Autodesk Fusion 360 part; units mm, degrees
(part 2 of 8)
  spline S328 degree 3 poles (150.3469, -208.3577) (147.0321, -208.3577) (145.9386, -207.6875) (144.7041, -207.6875) knots 0 0 0 0 1 1 1 1
  spline S329 degree 3 poles (144.7041, -207.6875) (143.8199, -207.6875) (143.538, -208.0049) (142.9741, -208.0049) knots 0 0 0 0 1 1 1 1
  spline S330 degree 3 poles (142.9741, -208.0049) (142.517, -208.0049) (142.2351, -207.5816) (142.0557, -206.9114) knots 0 0 0 0 1 1 1 1
  spline S331 degree 3 poles (142.0557, -206.9114) (141.9147, -206.3821) (140.787, -201.1963) (140.787, -200.9144) knots 0 0 0 0 1 1 1 1
  spline S332 degree 3 poles (140.787, -200.9144) (140.787, -200.632) (141.5644, -199.8913) (141.9873, -199.8913) knots 0 0 0 0 1 1 1 1
  spline S333 degree 3 poles (141.9873, -199.8913) (142.658, -199.8913) (145.6225, -205.8178) (150.7356, -205.8178) knots 0 0 0 0 1 1 1 1
  spline S334 degree 3 poles (150.7356, -205.8178) (152.7818, -205.8178) (154.0889, -204.9007) (154.0889, -203.4189) knots 0 0 0 0 1 1 1 1
  spline S335 degree 3 poles (154.0889, -203.4189) (154.0504, -199.3621) (141.4918, -199.9618) (141.4918, -191.1422) knots 0 0 0 0 1 1 1 1
  spline S336 degree 3 poles (177.5118, -204.8653) (177.5118, -206.3823) (179.4524, -206.2764) (179.4524, -206.8059) knots 0 0 0 0 1 1 1 1
  spline S337 degree 3 poles (179.4524, -206.8059) (179.4524, -207.2291) (179.0625, -208.0053) (178.7789, -208.0053) knots 0 0 0 0 1 1 1 1
  spline S338 degree 3 poles (178.7789, -208.0053) (177.4054, -207.9344) (175.6774, -207.8994) (173.9495, -207.8994) knots 0 0 0 0 1 1 1 1
  spline S339 degree 3 poles (173.9495, -207.8994) (172.2171, -207.8994) (170.5245, -207.9344) (169.1156, -208.0053) knots 0 0 0 0 1 1 1 1
  spline S340 degree 3 poles (169.1156, -208.0053) (168.832, -208.0053) (168.4775, -207.2291) (168.4775, -206.8059) knots 0 0 0 0 1 1 1 1
  spline S341 degree 3 poles (168.4775, -206.8059) (168.4775, -206.2765) (170.3827, -206.3823) (170.3827, -204.8653) knots 0 0 0 0 1 1 1 1
  line L72 (170.3827, -204.8653) -> (170.3827, -187.6147)
  spline S342 degree 3 poles (170.3827, -187.6147) (170.3827, -187.0853) (169.9618, -186.8385) (169.0092, -186.8385) knots 0 0 0 0 1 1 1 1
  spline S343 degree 3 poles (169.0092, -186.8385) (164.9507, -186.8385) (163.2582, -191.6715) (162.5891, -191.6715) knots 0 0 0 0 1 1 1 1
  spline S344 degree 3 poles (162.5891, -191.6715) (162.1638, -191.6715) (161.3884, -191.3188) (161.3884, -191.0011) knots 0 0 0 0 1 1 1 1
  spline S345 degree 3 poles (161.3884, -191.0011) (161.3884, -190.7189) (162.0574, -185.8154) (162.1283, -185.3568) knots 0 0 0 0 1 1 1 1
  spline S346 degree 3 poles (162.1283, -185.3568) (162.2701, -184.4397) (162.6246, -184.2243) (163.3645, -184.2633) knots 0 0 0 0 1 1 1 1
  spline S347 degree 3 poles (163.3645, -184.2633) (167.0331, -184.3338) (170.6663, -184.3692) (174.2995, -184.3692) knots 0 0 0 0 1 1 1 1
  spline S348 degree 3 poles (174.2995, -184.3692) (177.9327, -184.3692) (181.6058, -184.3338) (185.2389, -184.2633) knots 0 0 0 0 1 1 1 1
  spline S349 degree 3 poles (185.2389, -184.2633) (185.9434, -184.2244) (186.3688, -184.4397) (186.3688, -185.0746) knots 0 0 0 0 1 1 1 1
  spline S350 degree 3 poles (186.3688, -185.0746) (186.3688, -185.8154) (185.8415, -190.7189) (185.8415, -191.0011) knots 0 0 0 0 1 1 1 1
  spline S351 degree 3 poles (185.8415, -191.0011) (185.8415, -191.2834) (185.0617, -191.6715) (184.6408, -191.6715) knots 0 0 0 0 1 1 1 1
  spline S352 degree 3 poles (184.6408, -191.6715) (183.9718, -191.6715) (183.6882, -186.8385) (178.6416, -186.8385) knots 0 0 0 0 1 1 1 1
  spline S353 degree 3 poles (178.6416, -186.8385) (177.9327, -186.8385) (177.5118, -186.7326) (177.5118, -187.6147) knots 0 0 0 0 1 1 1 1
  line L73 (177.5118, -187.6147) -> (177.5118, -204.8653)
  spline S354 degree 3 poles (199.0684, -208.3577) (192.9284, -208.3577) (189.4714, -204.8651) (189.4714, -198.48) knots 0 0 0 0 1 1 1 1
  line L74 (189.4714, -198.48) -> (189.4714, -187.3674)
  spline S355 degree 3 poles (189.4714, -187.3674) (189.4714, -185.8857) (187.5667, -185.9915) (187.5667, -185.4274) knots 0 0 0 0 1 1 1 1
  spline S356 degree 3 poles (187.5667, -185.4274) (187.5667, -185.0039) (187.9192, -184.263) (188.2352, -184.263) knots 0 0 0 0 1 1 1 1
  spline S357 degree 3 poles (188.2352, -184.263) (189.65, -184.3336) (191.3395, -184.3688) (193.0703, -184.3688) knots 0 0 0 0 1 1 1 1
  spline S358 degree 3 poles (193.0703, -184.3688) (194.7644, -184.3688) (196.4906, -184.3336) (197.8688, -184.263) knots 0 0 0 0 1 1 1 1
  spline S359 degree 3 poles (197.8688, -184.263) (198.1481, -184.263) (198.5373, -185.0039) (198.5373, -185.4274) knots 0 0 0 0 1 1 1 1
  spline S360 degree 3 poles (198.5373, -185.4274) (198.5373, -185.9915) (196.5959, -185.8857) (196.5959, -187.3674) knots 0 0 0 0 1 1 1 1
  line L75 (196.5959, -187.3674) -> (196.5959, -198.9031)
  spline S361 degree 3 poles (196.5959, -198.9031) (196.5959, -202.9956) (198.3632, -205.1123) (201.3578, -205.1123) knots 0 0 0 0 1 1 1 1
  spline S362 degree 3 poles (201.3578, -205.1123) (204.3568, -205.1123) (206.1242, -202.9956) (206.1242, -198.9031) knots 0 0 0 0 1 1 1 1
  line L76 (206.1242, -198.9031) -> (206.1242, -187.3674)
  spline S363 degree 3 poles (206.1242, -187.3674) (206.1242, -185.8857) (204.1828, -185.9915) (204.1828, -185.4274) knots 0 0 0 0 1 1 1 1
  spline S364 degree 3 poles (204.1828, -185.4274) (204.1828, -185.0039) (204.572, -184.2241) (204.8513, -184.263) knots 0 0 0 0 1 1 1 1
  spline S365 degree 3 poles (204.8513, -184.263) (205.5564, -184.3336) (206.4767, -184.3688) (207.3925, -184.3688) knots 0 0 0 0 1 1 1 1
  spline S366 degree 3 poles (207.3925, -184.3688) (208.3082, -184.3688) (209.2285, -184.3336) (209.9337, -184.263) knots 0 0 0 0 1 1 1 1
  spline S367 degree 3 poles (209.9337, -184.263) (210.213, -184.2241) (210.4969, -185.0039) (210.4969, -185.4274) knots 0 0 0 0 1 1 1 1
  spline S368 degree 3 poles (210.4969, -185.4274) (210.4969, -185.9915) (208.6608, -185.8857) (208.6608, -187.3674) knots 0 0 0 0 1 1 1 1
  line L77 (208.6608, -187.3674) -> (208.6608, -198.48)
  spline S369 degree 3 poles (208.6608, -198.48) (208.6608, -204.8651) (205.2039, -208.3577) (199.0683, -208.3577) knots 0 0 0 0 1 1 1 1
  spline S370 degree 3 poles (213.773, -187.4032) (213.28, -185.9921) (211.6589, -186.0272) (211.6589, -185.4631) knots 0 0 0 0 1 1 1 1
  spline S371 degree 3 poles (211.6589, -185.4631) (211.6589, -185.0398) (212.0476, -184.2989) (212.3272, -184.2989) knots 0 0 0 0 1 1 1 1
  spline S372 degree 3 poles (212.3272, -184.2989) (213.7398, -184.3695) (215.5743, -184.4008) (217.4087, -184.4008) knots 0 0 0 0 1 1 1 1
  spline S373 degree 3 poles (217.4087, -184.4008) (219.2432, -184.4008) (221.0776, -184.3695) (222.4854, -184.2989) knots 0 0 0 0 1 1 1 1
  spline S374 degree 3 poles (222.4854, -184.2989) (222.7698, -184.2989) (223.1206, -185.0398) (223.1206, -185.4631) knots 0 0 0 0 1 1 1 1
  spline S375 degree 3 poles (223.1206, -185.4631) (223.1206, -186.0272) (220.9022, -185.9921) (221.3952, -187.4032) knots 0 0 0 0 1 1 1 1
  line L78 (226.652, -202.5727) -> (231.9089, -187.4032)
  spline S376 degree 3 poles (231.9089, -187.4032) (232.4019, -185.9921) (230.1787, -186.0272) (230.1787, -185.4631) knots 0 0 0 0 1 1 1 1
  spline S377 degree 3 poles (230.1787, -185.4631) (230.1787, -185.0398) (230.5295, -184.2633) (230.8139, -184.2989) knots 0 0 0 0 1 1 1 1
  spline S378 degree 3 poles (230.8139, -184.2989) (231.378, -184.3695) (232.4351, -184.4008) (233.4921, -184.4008) knots 0 0 0 0 1 1 1 1
  spline S379 degree 3 poles (233.4921, -184.4008) (234.554, -184.4008) (235.611, -184.3695) (236.1419, -184.2989) knots 0 0 0 0 1 1 1 1
  spline S380 degree 3 poles (236.1419, -184.2989) (236.4216, -184.2633) (236.8103, -185.0398) (236.8103, -185.4631) knots 0 0 0 0 1 1 1 1
  spline S381 degree 3 poles (236.8103, -185.4631) (236.8103, -186.0272) (235.1891, -185.9921) (234.6914, -187.4032) knots 0 0 0 0 1 1 1 1
  line L79 (234.6914, -187.4032) -> (227.4626, -208.0054)
  spline S382 degree 3 poles (227.4626, -208.0054) (226.2634, -207.9348) (225.2395, -207.8997) (224.2535, -207.8997) knots 0 0 0 0 1 1 1 1
  spline S383 degree 3 poles (224.2535, -207.8997) (223.2297, -207.8997) (222.239, -207.9348) (221.0065, -208.0054) knots 0 0 0 0 1 1 1 1
  line L80 (221.0065, -208.0054) -> (213.773, -187.4032)
  spline S384 degree 3 poles (250.2557, -207.8993) (249.2341, -207.8993) (248.2426, -207.9343) (247.0108, -208.0049) knots 0 0 0 0 1 1 1 1
  line L81 (247.0108, -208.0049) -> (239.7799, -187.4026)
  spline S385 degree 3 poles (239.7799, -187.4026) (239.2842, -185.9914) (237.6618, -186.027) (237.6618, -185.4627) knots 0 0 0 0 1 1 1 1
  spline S386 degree 3 poles (237.6618, -185.4627) (237.6618, -185.039) (238.0474, -184.2984) (238.3328, -184.2984) knots 0 0 0 0 1 1 1 1
  spline S387 degree 3 poles (238.3328, -184.2984) (239.7399, -184.369) (241.5777, -184.4006) (243.4104, -184.4006) knots 0 0 0 0 1 1 1 1
  spline S388 degree 3 poles (243.4104, -184.4006) (245.2432, -184.4006) (247.0809, -184.369) (248.4931, -184.2984) knots 0 0 0 0 1 1 1 1
  spline S389 degree 3 poles (248.4931, -184.2984) (248.7735, -184.2984) (249.124, -185.039) (249.124, -185.4627) knots 0 0 0 0 1 1 1 1
  spline S390 degree 3 poles (249.124, -185.4627) (249.124, -186.027) (246.9057, -185.9914) (247.3964, -187.4026) knots 0 0 0 0 1 1 1 1
  line L82 (247.3964, -187.4026) -> (252.5841, -202.3254)
  spline S391 degree 3 poles (252.5841, -202.3254) (254.2066, -197.5978) (257.9472, -189.8723) (257.3463, -187.4026) knots 0 0 0 0 1 1 1 1
  spline S392 degree 3 poles (257.3463, -187.4026) (256.8505, -185.9914) (255.2632, -186.027) (255.2632, -185.4627) knots 0 0 0 0 1 1 1 1
  spline S393 degree 3 poles (255.2632, -185.4627) (255.2632, -185.039) (255.6187, -184.2984) (255.8991, -184.2984) knots 0 0 0 0 1 1 1 1
  spline S394 degree 3 poles (255.8991, -184.2984) (257.3112, -184.369) (259.144, -184.4006) (260.9817, -184.4006) knots 0 0 0 0 1 1 1 1
  spline S395 degree 3 poles (260.9817, -184.4006) (262.8495, -184.4006) (264.6823, -184.369) (266.0594, -184.2984) knots 0 0 0 0 1 1 1 1
  spline S396 degree 3 poles (266.0594, -184.2984) (266.3398, -184.2984) (266.7304, -185.039) (266.7304, -185.4627) knots 0 0 0 0 1 1 1 1
  spline S397 degree 3 poles (266.7304, -185.4627) (266.7304, -186.027) (264.472, -185.9914) (264.9677, -187.4381) knots 0 0 0 0 1 1 1 1
  line L83 (264.9677, -187.4381) -> (270.2206, -202.5723)
  line L84 (270.2206, -202.5723) -> (275.4785, -187.4381)
  spline S398 degree 3 poles (275.4785, -187.4381) (275.9743, -185.9914) (273.7509, -186.027) (273.7509, -185.4627) knots 0 0 0 0 1 1 1 1
  spline S399 degree 3 poles (273.7509, -185.4627) (273.7509, -185.039) (274.1365, -184.2629) (274.4219, -184.2984) knots 0 0 0 0 1 1 1 1
  spline S400 degree 3 poles (274.4219, -184.2984) (274.9477, -184.369) (276.0093, -184.4006) (277.0659, -184.4006) knots 0 0 0 0 1 1 1 1
  spline S401 degree 3 poles (277.0659, -184.4006) (278.1225, -184.4006) (279.1841, -184.369) (279.7099, -184.2984) knots 0 0 0 0 1 1 1 1
  spline S402 degree 3 poles (279.7099, -184.2984) (280.0353, -184.2629) (280.3859, -185.039) (280.3859, -185.4627) knots 0 0 0 0 1 1 1 1
  spline S403 degree 3 poles (280.3859, -185.4627) (280.3859, -186.027) (278.7985, -185.9914) (278.3028, -187.4026) knots 0 0 0 0 1 1 1 1
  line L85 (278.3028, -187.4026) -> (271.0319, -208.0049)
  spline S404 degree 3 poles (271.0319, -208.0049) (269.835, -207.9343) (268.8135, -207.8993) (267.8221, -207.8993) knots 0 0 0 0 1 1 1 1
  spline S405 degree 3 poles (267.8221, -207.8993) (266.8005, -207.8993) (265.8141, -207.9343) (264.5772, -208.0049) knots 0 0 0 0 1 1 1 1
  line L86 (264.5772, -208.0049) -> (259.1791, -192.6239)
  spline S406 degree 3 poles (259.1791, -192.6239) (257.4866, -198.1627) (254.0665, -204.6534) (253.4656, -208.0049) knots 0 0 0 0 1 1 1 1
  spline S407 degree 3 poles (253.4656, -208.0049) (252.2638, -207.9343) (251.2422, -207.8993) (250.2558, -207.8993) knots 0 0 0 0 1 1 1 1
  line L87 (296.6782, -193.2941) -> (300.5229, -187.4382)
  spline S408 degree 3 poles (300.5229, -187.4382) (301.3342, -186.168) (299.324, -185.9918) (299.324, -185.4275) knots 0 0 0 0 1 1 1 1
  spline S409 degree 3 poles (299.324, -185.4275) (299.324, -185.0042) (299.8201, -184.2244) (300.0992, -184.2632) knots 0 0 0 0 1 1 1 1
  spline S410 degree 3 poles (300.0992, -184.2632) (300.6314, -184.334) (301.6185, -184.3691) (302.6055, -184.3691) knots 0 0 0 0 1 1 1 1
  spline S411 degree 3 poles (302.6055, -184.3691) (303.5925, -184.3691) (304.5795, -184.334) (305.1118, -184.2632) knots 0 0 0 0 1 1 1 1
  spline S412 degree 3 poles (305.1118, -184.2632) (305.3908, -184.2244) (305.7784, -185.0042) (305.7784, -185.4275) knots 0 0 0 0 1 1 1 1
  spline S413 degree 3 poles (305.7784, -185.4275) (305.7784, -185.9918) (304.5485, -186.168) (303.701, -187.4382) knots 0 0 0 0 1 1 1 1
  line L88 (303.701, -187.4382) -> (298.1975, -195.6227)
  line L89 (298.1975, -195.6227) -> (304.2281, -204.8655)
  spline S414 degree 3 poles (304.2281, -204.8655) (305.0394, -206.1352) (306.4864, -206.2763) (306.4864, -206.8411) knots 0 0 0 0 1 1 1 1
  spline S415 degree 3 poles (306.4864, -206.8411) (306.4864, -207.2643) (306.0988, -208.0053) (305.8146, -208.0053) knots 0 0 0 0 1 1 1 1
  spline S416 degree 3 poles (305.8146, -208.0053) (304.44, -207.9346) (302.3574, -207.8994) (300.3111, -207.8994) knots 0 0 0 0 1 1 1 1
  spline S417 degree 3 poles (300.3111, -207.8994) (298.2337, -207.8994) (296.1873, -207.9346) (294.7765, -208.0053) knots 0 0 0 0 1 1 1 1
  spline S418 degree 3 poles (294.7765, -208.0053) (294.4923, -208.0053) (294.1048, -207.2643) (294.1048, -206.8411) knots 0 0 0 0 1 1 1 1
  spline S419 degree 3 poles (294.1048, -206.8411) (294.1048, -206.2763) (296.5026, -206.1352) (295.6912, -204.8655) knots 0 0 0 0 1 1 1 1
  line L90 (295.6912, -204.8655) -> (291.1075, -197.8804)
  line L91 (291.1075, -197.8804) -> (286.591, -204.8304)
  spline S420 degree 3 poles (286.591, -204.8304) (285.7435, -206.1) (287.7537, -206.2763) (287.7537, -206.8054) knots 0 0 0 0 1 1 1 1
  spline S421 degree 3 poles (287.7537, -206.8054) (287.7537, -207.2292) (287.2576, -208.0405) (286.9786, -208.0053) knots 0 0 0 0 1 1 1 1
  spline S422 degree 3 poles (286.9786, -208.0053) (286.4463, -207.9345) (285.4593, -207.8994) (284.4723, -207.8994) knots 0 0 0 0 1 1 1 1
  spline S423 degree 3 poles (284.4723, -207.8994) (283.4853, -207.8994) (282.4982, -207.9345) (281.966, -208.0053) knots 0 0 0 0 1 1 1 1
  spline S424 degree 3 poles (281.966, -208.0053) (281.6869, -208.0405) (281.2993, -207.2292) (281.2993, -206.8054) knots 0 0 0 0 1 1 1 1
  spline S425 degree 3 poles (281.2993, -206.8054) (281.2993, -206.2763) (282.5344, -206.1) (283.3819, -204.8304) knots 0 0 0 0 1 1 1 1
  line L92 (283.3819, -204.8304) -> (289.6244, -195.5875)
  line L93 (289.6244, -195.5875) -> (284.2966, -187.3674)
  spline S426 degree 3 poles (284.2966, -187.3674) (283.449, -186.0977) (282.0021, -185.9918) (282.0021, -185.4275) knots 0 0 0 0 1 1 1 1
  spline S427 degree 3 poles (282.0021, -185.4275) (282.0021, -185.0042) (282.3897, -184.2244) (282.6739, -184.2632) knots 0 0 0 0 1 1 1 1
  spline S428 degree 3 poles (282.6739, -184.2632) (284.0847, -184.334) (286.1311, -184.3691) (288.2136, -184.3691) knots 0 0 0 0 1 1 1 1
  spline S429 degree 3 poles (288.2136, -184.3691) (290.26, -184.3691) (292.3426, -184.334) (293.7171, -184.2632) knots 0 0 0 0 1 1 1 1
  spline S430 degree 3 poles (293.7171, -184.2632) (293.9962, -184.2244) (294.3838, -185.0042) (294.3838, -185.4275) knots 0 0 0 0 1 1 1 1
  spline S431 degree 3 poles (294.3838, -185.4275) (294.3838, -185.9566) (291.986, -186.0977) (292.8335, -187.3674) knots 0 0 0 0 1 1 1 1
  line L94 (292.8335, -187.3674) -> (296.6782, -193.2941)
  spline S432 degree 3 poles (309.125, -187.3682) (308.418, -186.0626) (307.3601, -185.9919) (307.3601, -185.4279) knots 0 0 0 0 1 1 1 1
  spline S433 degree 3 poles (307.3601, -185.4279) (307.3601, -185.0042) (307.7482, -184.2637) (308.0299, -184.2637) knots 0 0 0 0 1 1 1 1
  spline S434 degree 3 poles (308.0299, -184.2637) (309.4439, -184.3339) (311.2088, -184.3695) (312.9737, -184.3695) knots 0 0 0 0 1 1 1 1
  spline S435 degree 3 poles (312.9737, -184.3695) (314.7704, -184.3695) (316.5353, -184.3339) (317.9493, -184.2637) knots 0 0 0 0 1 1 1 1
  spline S436 degree 3 poles (317.9493, -184.2637) (318.231, -184.2637) (318.5819, -185.0042) (318.5819, -185.4279) knots 0 0 0 0 1 1 1 1
  spline S437 degree 3 poles (318.5819, -185.4279) (318.5819, -185.9919) (316.4981, -186.0626) (317.2051, -187.4032) knots 0 0 0 0 1 1 1 1
  line L95 (317.2051, -187.4032) -> (321.5854, -195.9756)
  line L96 (321.5854, -195.9756) -> (325.955, -187.4032)
  spline S438 degree 3 poles (325.955, -187.4032) (326.662, -186.0626) (324.5836, -185.9919) (324.5836, -185.4279) knots 0 0 0 0 1 1 1 1
  spline S439 degree 3 poles (324.5836, -185.4279) (324.5836, -185.0042) (324.9344, -184.2244) (325.2162, -184.2637) knots 0 0 0 0 1 1 1 1
  spline S440 degree 3 poles (325.2162, -184.2637) (325.7796, -184.3339) (326.6993, -184.3695) (327.6136, -184.3695) knots 0 0 0 0 1 1 1 1
  spline S441 degree 3 poles (327.6136, -184.3695) (328.5332, -184.3695) (329.4476, -184.3339) (329.9792, -184.2637) knots 0 0 0 0 1 1 1 1
  spline S442 degree 3 poles (329.9792, -184.2637) (330.2609, -184.2244) (330.6489, -185.0042) (330.6489, -185.4279) knots 0 0 0 0 1 1 1 1
  spline S443 degree 3 poles (330.6489, -185.4279) (330.6489, -185.9919) (329.5911, -186.0626) (328.8841, -187.4032) knots 0 0 0 0 1 1 1 1
  line L97 (328.8841, -187.4032) -> (322.5689, -199.7855)
  line L98 (322.5689, -199.7855) -> (322.5689, -204.8659)
  spline S444 degree 3 poles (322.5689, -204.8659) (322.5689, -206.3825) (324.5092, -206.2767) (324.5092, -206.8412) knots 0 0 0 0 1 1 1 1
  spline S445 degree 3 poles (324.5092, -206.8412) (324.5092, -207.2644) (324.1211, -208.0054) (323.8394, -208.0054) knots 0 0 0 0 1 1 1 1
  spline S446 degree 3 poles (323.8394, -208.0054) (322.4626, -207.9347) (320.7349, -207.8996) (319.0072, -207.8996) knots 0 0 0 0 1 1 1 1
  spline S447 degree 3 poles (319.0072, -207.8996) (317.2796, -207.8996) (315.5838, -207.9347) (314.1698, -208.0054) knots 0 0 0 0 1 1 1 1
  spline S448 degree 3 poles (314.1698, -208.0054) (313.8881, -208.0054) (313.5372, -207.2644) (313.5372, -206.8412) knots 0 0 0 0 1 1 1 1
  spline S449 degree 3 poles (313.5372, -206.8412) (313.5372, -206.2767) (315.4403, -206.3825) (315.4403, -204.8659) knots 0 0 0 0 1 1 1 1
  line L99 (315.4403, -204.8659) -> (315.4403, -199.7855)
  line L100 (315.4403, -199.7855) -> (309.125, -187.3682)
  spline S450 degree 3 poles (350.616, -184.2631) (350.8992, -184.2245) (351.2859, -185.0039) (351.2859, -185.4277) knots 0 0 0 0 1 1 1 1
  spline S451 degree 3 poles (351.2859, -185.4277) (351.2859, -185.9565) (351.3567, -186.0976) (350.5833, -187.3678) knots 0 0 0 0 1 1 1 1
  line L101 (350.5833, -187.3678) -> (340.3868, -204.2655)
  spline S452 degree 3 poles (340.3868, -204.2655) (339.9238, -205.0417) (340.7735, -205.3946) (342.5765, -205.3946) knots 0 0 0 0 1 1 1 1
  spline S453 degree 3 poles (342.5765, -205.3946) (348.7477, -205.3946) (350.1584, -201.3024) (350.8284, -201.3024) knots 0 0 0 0 1 1 1 1
  spline S454 degree 3 poles (350.8284, -201.3024) (351.2532, -201.3024) (351.994, -201.6554) (351.994, -201.9375) knots 0 0 0 0 1 1 1 1
  spline S455 degree 3 poles (351.994, -201.9375) (351.994, -202.2197) (351.0408, -206.4529) (350.8992, -206.9824) knots 0 0 0 0 1 1 1 1
  spline S456 degree 3 poles (350.8992, -206.9824) (350.6868, -207.7934) (350.3709, -208.0407) (349.6683, -208.0053) knots 0 0 0 0 1 1 1 1
  spline S457 degree 3 poles (349.6683, -208.0053) (347.1954, -207.9345) (343.8783, -207.8996) (340.5939, -207.8996) knots 0 0 0 0 1 1 1 1
  spline S458 degree 3 poles (340.5939, -207.8996) (337.2822, -207.8996) (333.9651, -207.9345) (331.4923, -208.0053) knots 0 0 0 0 1 1 1 1
  spline S459 degree 3 poles (331.4923, -208.0053) (331.1764, -208.0053) (330.8223, -207.2645) (330.8223, -206.8407) knots 0 0 0 0 1 1 1 1
  spline S460 degree 3 poles (330.8223, -206.8407) (330.8223, -206.2765) (330.8931, -206.1708) (331.672, -204.9006) knots 0 0 0 0 1 1 1 1
  line L102 (331.672, -204.9006) -> (342.1136, -187.6146)
  spline S461 degree 3 poles (342.1136, -187.6146) (342.3587, -187.1559) (341.6887, -186.8384) (340.2072, -186.8384) knots 0 0 0 0 1 1 1 1
  spline S462 degree 3 poles (340.2072, -186.8384) (334.9184, -186.8384) (333.012, -191.1425) (332.342, -191.1425) knots 0 0 0 0 1 1 1 1
  spline S463 degree 3 poles (332.342, -191.1425) (331.9171, -191.1425) (331.1763, -190.7541) (331.1763, -190.472) knots 0 0 0 0 1 1 1 1
  spline S464 degree 3 poles (331.1763, -190.472) (331.1763, -190.1898) (331.9879, -185.8155) (332.0914, -185.2512) knots 0 0 0 0 1 1 1 1
  spline S465 degree 3 poles (332.0914, -185.2512) (332.2003, -184.4396) (332.587, -184.2245) (333.2951, -184.2631) knots 0 0 0 0 1 1 1 1
  spline S466 degree 3 poles (333.2951, -184.2631) (338.2299, -184.3693) (345.6812, -184.4009) (350.616, -184.2631) knots 0 0 0 0 1 1 1 1
  line L103 (212.3272, -184.2989) -> (222.4854, -184.2989)
  spline S467 degree 5 poles (222.4854, -184.2989) (222.5535, -184.3209) (222.6812, -184.3676) (222.8473, -184.4461) (223.0168, -184.5677) (223.1369, -184.7495) (223.1591, -184.9634) (223.0788, -185.2107) (222.899, -185.4905) (222.6281, -185.8) (222.275, -186.1363) (221.9333, -186.4247) (221.6459, -186.6511) (221.4408, -186.8065) (221.3348, -186.8853) knots 0 0 0 0 0 0 0.1 0.2 0.3 0.4 0.5 0.6 0.7 0.8 0.9 1 1 1 1 1 1
  line L104 (221.3348, -186.8853) -> (226.652, -202.5727)
  line L105 (226.652, -202.5727) -> (231.9089, -187.4032)
  line L106 (221.3348, -186.8853) -> (226.652, -202.5727)
  line L107 (230.8139, -184.2989) -> (236.1419, -184.2989)
  line L108 (234.6914, -187.4032) -> (227.4626, -208.0054)
  line L109 (227.4626, -208.0054) -> (221.0065, -208.0054)
  line L110 (221.0065, -208.0054) -> (213.773, -187.4032)
  spline S468 degree 5 poles (213.773, -187.4032) (213.7536, -187.3475) (213.7109, -187.2382) (213.6354, -187.0807) (213.5118, -186.8839) (213.3192, -186.66) (213.0903, -186.4578) (212.8307, -186.2759) (212.5511, -186.1111) (212.2697, -185.9572) (212.0091, -185.8066) (211.7935, -185.6509) (211.6457, -185.4823) (211.5834, -185.2945) (211.6162, -185.0839) (211.7474, -184.8489) (211.9311, -184.6411) (212.1123, -184.4742) (212.2524, -184.3581) (212.3272, -184.2989) knots 0 0 0 0 0 0 0.066667 0.133333 0.2 0.266667 0.333333 0.4 0.466667 0.533333 0.6 0.666667 0.733333 0.8 0.866667 0.933333 1 1 1 1 1 1
  line L111 (238.4392, -186.0672) -> (247.0108, -208.0049)
  line L112 (247.0108, -208.0049) -> (253.4656, -208.0049)
  line L113 (64.1685, -187.3677) -> (64.1685, -204.9006)
  line L114 (71.2939, -199.9972) -> (71.2939, -204.9006)
  ellipse E0 centre (101, -197) end of major axis (101, -183.912) minor radius 11.3829
  line L115 (101, -210.088) -> (101, -183.912)
  line L116 (112.3829, -197) -> (89.6171, -197)
  point P0 (223.1206, -185.0409)
  point P1 (212.7978, -186.2622)
  constraint coincident S375 S467.end
  constraint coincident S370 P1
  constraint coincident S385 L111.start
  constraint coincident E0 L115.start
  constraint coincident E0 L115.end
  constraint coincident E0 L116.start
  constraint coincident E0 L116.end
  constraint vertical L115
extrude "Extrude1" add sketch "Sketch1" along normal blind 1 contours S0 S1 S2 S3 S4 S5 L3 S6 S7 S8 S9 L4 S10 S11 S12 S13 S14 S15 L5 L6 L7 | S22 S23 S24 S25 S26 L12 S27 S28 S29 S30 S31 S32 S33 | S34 S35 S36 S37 S38 S39 S40 S41 S42 S43 S44 S45 S46 | S51 S52 S53 L14 S54 S55 S56 S57 S58 S59 S60 | L15 S61 S62 S63 S64 S65 L16 L17 S66 S67 S68 S69 S70 S71 S72 S73 S74 L18 S75 S76 S77 S78 S79 S80 S81 S82 S83 L19 | L20 S84 S85 S86 S87 S88 L21 L22 S89 S90 S91 S92 S93 S94 L23 S95 S96 S97 S98 S99 S100 S101 S102 S103 L24 | S104 S105 S106 S107 S108 S109 S110 S111 S112 S113 L25 S114 S115 S116 S117 S118 S119 S120 S121 S122 L26 S123 S124 | L27 L28 S125 S126 S127 S128 S129 S130 L29 S131 S132 S133 S134 S135 S136 L30 L31 L32 S137 S138 S139 S140 S141 S142 L33 S143 S144 S145 S146 S147 S148 L34 | S149 S150 S151 S152 S153 S154 L35 S155 S156 S157 S158 S159 S160 L36 | S161 S162 S163 L37 S164 S165 S166 S167 S168 S169 L38 S170 | L39 S171 S172 S173 S174 S175 S176 L40 L41 S177 S178 S179 S180 S181 S182 L42 L43 L44 S183 S184 S185 S186 S187 S188 L45 S189 S190 S191 S192 S193 S194 L46 | S195 S196 S197 S198 S199 S200 S201 S202 S203 L47 S204 S205 S206 S207 S208 S209 L48 | S210 S211 S212 L49 L50 S213 S214 S215 S216 L51 S217 S218 S219 S220 S221 S222 L52 L53 S223 S224 L54 L55 S225 S226 S227 S228 S229 S230 L56 S231 | S232 S233 S234 L57 L58 S235 S236 S237 S238 S239 S240 L59 S241 S242 S243 S244 L60 L61 S245 S246 S247 S248 S249 S250 L62 S251 | S256 S257 S258 S259 | S264 S265 S266 S267 S268 S269 L64 S270 S271 S272 S273 S274 S275 S276 L65 L113 L114 | S277 S280 S297 E0 L115 L116 | S277 S278 S279 E0 L115 L116 | S280 S281 S282 E0 L115 L116 | S279 S280 S294 S295 E0 L115 L116 | S282 S283 S284 S285 S286 S287 S288 S289 S290 S291 S292 S293 S294 E0 | S301 S302 S303 S304 S305 S306 S307 S308 S309 S310 S311 L68 L69 L70 S312 S313 S314 S315 S316 S317 L71 | S318 S319 S320 S321 S322 S323 S324 S325 S326 S327 S328 S329 S330 S331 S332 S333 S334 S335 | S336 S337 S338 S339 S340 S341 L72 S342 S343 S344 S345 S346 S347 S348 S349 S350 S351 S352 S353 L73 | S354 L74 S355 S356 S357 S358 S359 S360 L75 S361 S362 L76 S363 S364 S365 S366 S367 S368 L77 S369 | S370 S371 S372 S373 S374 S375 L78 S376 S377 S378 S379 S380 S381 L79 S382 S383 L80 S467 L104 L105 L106 L108 L110 S468 | S384 S407 L112 | S384 L81 S385 S386 S387 S388 S389 S390 L82 S391 S392 S393 S394 S395 S396 S397 L83 L84 S398 S399 S400 S401 S402 S403 L85 S404 S405 L86 S406 S407 | L87 S408 S409 S410 S411 S412 S413 L88 L89 S414 S415 S416 S417 S418 S419 L90 L91 S420 S421 S422 S423 S424 S425 L92 L93 S426 S427 S428 S429 S430 S431 L94 | S432 S433 S434 S435 S436 S437 L95 L96 S438 S439 S440 S441 S442 S443 L97 L98 S444 S445 S446 S447 S448 S449 L99 L100 | S450 S451 L101 S452 S453 S454 S455 S456 S457 S458 S459 S460 L102 S461 S462 S463 S464 S465 S466 makes body 1 at (-221.8465, -188.4448, 0) makes body 2 at (-130.7268, -198.9655, 0) makes body 3 at (-67.7953, -195.9754, 0) makes body 4 at (55.5894, -193.7499, 0) makes body 5 at (149.7663, -197.1011, 0) makes body 6 at (338.0575, -198.9269, 0) makes body 7 at (246.4583, -199.2443, 0) makes body 8 at (220.4772, -199.3271, 0) makes body 9 at (118.7535, -195.8921, 0) makes body 10 at (23.5976, -199.8089, 0) makes body 11 at (-80.2131, -201.0084, 0) makes body 12 at (-165.1937, -195.799, 0) makes body 13 at (-264.0048, -196.3635, 0) makes body 14 at (-213.8759, -198.974, 0) makes body 15 at (-120.6379, -196.3399, 0) makes body 16 at (-39.7142, -198.8447, 0) makes body 17 at (66.5436, -196.5986, 0) makes body 18 at (172.7591, -193.3649, 0) makes body 19 at (313.9235, -191.519, 0) makes body 20 at (299.3723, -201.7846, 0) makes body 21 at (194.2211, -194.9168, 0) makes body 22 at (100.8692, -210.7763, 0) makes body 23 at (-12.0094, -193.2355, 0) makes body 24 at (-90.252, -199.0328, 0) makes body 25 at (-187.2421, -196.3987, 0) makes body 26 at (-277.1265, -196.2811, 0)
move_body "Move1" bodies 4 24 26 25 13 1 16 2 10 3 7 11 14 22 18 19 20 17 5 6 9 15 21 12 8 23 to x (1, 0, 0) y (0, 1, 0) z (0, 0, 1) at (-33.1187, 193.7133, 0)
scale "Scale1" factor 0.5 about (-120.9953, 6.3457, 0) bodies 22 23 15 11 7 5 21 26 9 14 10 1 3 25 17 12 20 18 8 6 19 4 13 2 16 24
scale "Scale2" factor 1.5 about (-40.4942, 1.107, 0) bodies 7 19 26 1 13 16 2 23 5 21 4 15 6 12 14 22 20 3 18 11 25 8 24 9 10 17
sketch "Sketch2" plane through (0, 0, 0.75) normal (0, 0, 1) x (-1, 0, 0)
  line L0 (306.2614, -0.2867) -> (311.1567, -0.3132)
  line L1 (311.1567, -0.3132) -> (308.7223, -7.2188)
  line L2 (308.7223, -7.2188) -> (306.2614, -0.2867)
  line L3 (311.8446, 1.6183) -> (305.6267, 1.5654)
  line L4 (305.6267, 1.5654) -> (304.7004, 4.1318)
  spline S0 degree 3 poles (304.7004, 4.1318) (304.3299, 5.2166) (306.0235, 5.1902) (306.0235, 5.587) knots -1 -1 -1 -1 0 0 0 0
  spline S1 degree 3 poles (306.0235, 5.587) (306.0235, 5.9045) (305.7322, 6.4866) (305.5206, 6.4866) knots -1 -1 -1 -1 0 0 0 0
  spline S2 degree 3 poles (305.5206, 6.4866) (304.4622, 6.4337) (303.1129, 6.4072) (301.737, 6.4072) knots -1 -1 -1 -1 0 0 0 0
  spline S3 degree 3 poles (301.737, 6.4072) (300.3609, 6.4072) (298.9851, 6.4337) (297.9265, 6.4866) knots -1 -1 -1 -1 0 0 0 0
  spline S4 degree 3 poles (297.9265, 6.4866) (297.7151, 6.4866) (297.4505, 5.9045) (297.4505, 5.587) knots -1 -1 -1 -1 0 0 0 0
  spline S5 degree 3 poles (297.4505, 5.587) (297.4505, 5.1902) (298.6411, 5.2166) (299.0115, 4.1318) knots -1 -1 -1 -1 0 0 0 0
  line L5 (299.0115, 4.1318) -> (304.277, -10.6848)
  spline S6 degree 3 poles (304.277, -10.6848) (304.4358, -11.1346) (304.7003, -11.2934) (305.5999, -11.2934) knots -1 -1 -1 -1 0 0 0 0
  spline S7 degree 3 poles (305.5999, -11.2934) (306.4998, -11.2934) (308.5106, -11.1346) (310.3894, -11.2934) knots -1 -1 -1 -1 0 0 0 0
  spline S8 degree 3 poles (310.3894, -11.2934) (310.6011, -11.3225) (310.8919, -10.7378) (310.8919, -10.4203) knots -1 -1 -1 -1 0 0 0 0
  spline S9 degree 3 poles (310.8919, -10.4203) (310.8919, -10.1557) (310.3627, -10.0234) (309.9129, -9.6794) knots -1 -1 -1 -1 0 0 0 0
  line L6 (309.9129, -9.6794) -> (314.8347, 4.1318)
  spline S10 degree 3 poles (314.8347, 4.1318) (315.2051, 5.1902) (316.3957, 5.1902) (316.3957, 5.587) knots -1 -1 -1 -1 0 0 0 0
  spline S11 degree 3 poles (316.3957, 5.587) (316.3957, 5.9045) (316.1311, 6.5131) (315.893, 6.4866) knots -1 -1 -1 -1 0 0 0 0
  spline S12 degree 3 poles (315.893, 6.4866) (315.4961, 6.4337) (314.7024, 6.4072) (313.9086, 6.4072) knots -1 -1 -1 -1 0 0 0 0
  spline S13 degree 3 poles (313.9086, 6.4072) (313.1149, 6.4072) (312.3209, 6.4337) (311.924, 6.4866) knots -1 -1 -1 -1 0 0 0 0
  spline S14 degree 3 poles (311.924, 6.4866) (311.7123, 6.5131) (311.4213, 5.9045) (311.4213, 5.587) knots -1 -1 -1 -1 0 0 0 0
  spline S15 degree 3 poles (311.4213, 5.587) (311.4213, 5.1902) (313.1411, 5.2166) (312.7442, 4.1318) knots -1 -1 -1 -1 0 0 0 0
  line L7 (312.7442, 4.1318) -> (311.8446, 1.6183)
  spline S16 degree 3 poles (-17.7132, 4.8726) (-19.2478, 4.8726) (-20.2282, 4.1848) (-20.2282, 3.0734) knots 0 0 0 0 1 1 1 1
  spline S17 degree 3 poles (-20.2282, 3.0734) (-20.2282, 4.1848) (-19.2478, 4.8726) (-17.7132, 4.8726) knots -1 -1 -1 -1 0 0 0 0
  spline S18 degree 3 poles (309.9129, -9.6794) (310.3627, -10.0234) (310.8919, -10.1557) (310.8919, -10.4203) knots 0 0 0 0 1 1 1 1
  spline S19 degree 3 poles (310.8919, -10.4203) (310.8919, -10.1557) (310.3627, -10.0234) (309.9129, -9.6794) knots -1 -1 -1 -1 0 0 0 0
  spline S20 degree 3 poles (306.0235, 5.587) (306.0235, 5.1902) (304.3299, 5.2166) (304.7004, 4.1318) knots 0 0 0 0 1 1 1 1
  spline S21 degree 3 poles (304.7004, 4.1318) (304.3299, 5.2166) (306.0235, 5.1902) (306.0235, 5.587) knots -1 -1 -1 -1 0 0 0 0
  line L8 (306.2614, -0.2867) -> (311.1567, -0.3132)
  line L9 (311.1567, -0.3132) -> (306.2614, -0.2867)
  spline S22 degree 3 poles (-13.1896, 6.2749) (-12.5264, 6.2749) (-12.315, 6.5129) (-11.8921, 6.5129) knots 0 0 0 0 1 1 1 1
  spline S23 degree 3 poles (-11.8921, 6.5129) (-12.315, 6.5129) (-12.5264, 6.2749) (-13.1896, 6.2749) knots -1 -1 -1 -1 0 0 0 0
  spline S24 degree 3 poles (-20.2282, 3.0734) (-20.2282, 4.1848) (-19.2478, 4.8726) (-17.7132, 4.8726) knots -1 -1 -1 -1 0 0 0 0
  spline S25 degree 3 poles (-17.7132, 4.8726) (-13.8784, 4.8726) (-11.655, 0.4277) (-11.152, 0.4277) knots -1 -1 -1 -1 0 0 0 0
  spline S26 degree 3 poles (-11.152, 0.4277) (-10.8349, 0.4277) (-10.2518, 0.9833) (-10.2518, 1.195) knots -1 -1 -1 -1 0 0 0 0
  spline S27 degree 3 poles (-10.2518, 1.195) (-10.2518, 1.4065) (-11.0976, 5.2958) (-11.2033, 5.6928) knots -1 -1 -1 -1 0 0 0 0
  spline S28 degree 3 poles (-11.2033, 5.6928) (-11.3378, 6.1954) (-11.5493, 6.5129) (-11.8921, 6.5129) knots -1 -1 -1 -1 0 0 0 0
  spline S29 degree 3 poles (-11.8921, 6.5129) (-12.315, 6.5129) (-12.5264, 6.2749) (-13.1896, 6.2749) knots -1 -1 -1 -1 0 0 0 0
  spline S30 degree 3 poles (-13.1896, 6.2749) (-14.1155, 6.2749) (-14.9356, 6.7775) (-17.4217, 6.7775) knots -1 -1 -1 -1 0 0 0 0
  spline S31 degree 3 poles (-17.4217, 6.7775) (-22.2658, 6.7775) (-24.9921, 4.8197) (-24.9921, 1.3536) knots -1 -1 -1 -1 0 0 0 0
  spline S32 degree 3 poles (-24.9921, 1.3536) (-24.9921, -5.1022) (-15.6244, -4.5467) (-15.6244, -7.8539) knots -1 -1 -1 -1 0 0 0 0
  spline S33 degree 3 poles (-15.6244, -7.8539) (-15.6244, -8.8858) (-16.5759, -9.6531) (-17.8446, -9.6531) knots -1 -1 -1 -1 0 0 0 0
  spline S34 degree 3 poles (-17.8446, -9.6531) (-20.9682, -9.6531) (-23.0571, -5.7372) (-23.5601, -5.7372) knots -1 -1 -1 -1 0 0 0 0
  spline S35 degree 3 poles (-23.5601, -5.7372) (-23.8804, -5.7372) (-24.4347, -6.2927) (-24.4347, -6.5045) knots -1 -1 -1 -1 0 0 0 0
  spline S36 degree 3 poles (-24.4347, -6.5045) (-24.4347, -6.7163) (-23.8804, -10.0763) (-23.7491, -10.4733) knots -1 -1 -1 -1 0 0 0 0
  spline S37 degree 3 poles (-23.7491, -10.4733) (-23.6177, -10.976) (-23.4287, -11.2934) (-23.0859, -11.2934) knots -1 -1 -1 -1 0 0 0 0
  spline S38 degree 3 poles (-23.0859, -11.2934) (-22.6342, -11.2934) (-22.4483, -11.0288) (-21.7884, -11.0288) knots -1 -1 -1 -1 0 0 0 0
  spline S39 degree 3 poles (-21.7884, -11.0288) (-20.8625, -11.0288) (-19.8821, -11.5581) (-17.5018, -11.5581) knots -1 -1 -1 -1 0 0 0 0
  spline S40 degree 3 poles (-17.5018, -11.5581) (-13.401, -11.5581) (-10.7804, -9.4414) (-10.7804, -6.1341) knots -1 -1 -1 -1 0 0 0 0
  spline S41 degree 3 poles (-10.7804, -6.1341) (-10.7804, 0.4806) (-20.1993, 0.0308) (-20.2282, 3.0734) knots -1 -1 -1 -1 0 0 0 0
  line L10 (308.7223, -7.2188) -> (306.2614, -0.2867)
  line L11 (306.2614, -0.2867) -> (308.7223, -7.2188)
  spline S42 degree 3 poles (301.737, 6.4072) (303.1129, 6.4072) (304.4622, 6.4337) (305.5206, 6.4866) knots 0 0 0 0 1 1 1 1
  spline S43 degree 3 poles (305.5206, 6.4866) (304.4622, 6.4337) (303.1129, 6.4072) (301.737, 6.4072) knots -1 -1 -1 -1 0 0 0 0
  spline S44 degree 3 poles (297.9265, 6.4866) (298.9851, 6.4337) (300.3609, 6.4072) (301.737, 6.4072) knots 0 0 0 0 1 1 1 1
  spline S45 degree 3 poles (301.737, 6.4072) (300.3609, 6.4072) (298.9851, 6.4337) (297.9265, 6.4866) knots -1 -1 -1 -1 0 0 0 0
  spline S46 degree 3 poles (-10.7804, -6.1341) (-10.7804, -9.4414) (-13.401, -11.5581) (-17.5018, -11.5581) knots 0 0 0 0 1 1 1 1
  spline S47 degree 3 poles (-17.5018, -11.5581) (-13.401, -11.5581) (-10.7804, -9.4414) (-10.7804, -6.1341) knots -1 -1 -1 -1 0 0 0 0
  spline S48 degree 3 poles (-53.5645, -10.4202) (-53.5645, -9.9971) (-52.1084, -10.0765) (-52.1084, -8.9652) knots 0 0 0 0 1 1 1 1
  spline S49 degree 3 poles (-52.1084, -8.9652) (-52.1084, -10.0765) (-53.5645, -9.9971) (-53.5645, -10.4202) knots -1 -1 -1 -1 0 0 0 0
  line L12 (311.1567, -0.3132) -> (308.7223, -7.2188)
  line L13 (308.7223, -7.2188) -> (311.1567, -0.3132)
  spline S50 degree 3 poles (-23.5601, -5.7372) (-23.0571, -5.7372) (-20.9682, -9.6531) (-17.8446, -9.6531) knots 0 0 0 0 1 1 1 1
  spline S51 degree 3 poles (-17.8446, -9.6531) (-20.9682, -9.6531) (-23.0571, -5.7372) (-23.5601, -5.7372) knots -1 -1 -1 -1 0 0 0 0
  spline S52 degree 3 poles (315.893, 6.4866) (316.1311, 6.5131) (316.3957, 5.9045) (316.3957, 5.587) knots 0 0 0 0 1 1 1 1
  spline S53 degree 3 poles (316.3957, 5.587) (316.3957, 5.9045) (316.1311, 6.5131) (315.893, 6.4866) knots -1 -1 -1 -1 0 0 0 0
  spline S54 degree 3 poles (-57.7986, -10.4202) (-57.7986, -10.7379) (-58.0905, -11.3227) (-58.3, -11.2935) knots 0 0 0 0 1 1 1 1
  spline S55 degree 3 poles (-58.3, -11.2935) (-58.0905, -11.3227) (-57.7986, -10.7379) (-57.7986, -10.4202) knots -1 -1 -1 -1 0 0 0 0
  spline S56 degree 3 poles (305.5999, -11.2934) (304.7003, -11.2934) (304.4358, -11.1346) (304.277, -10.6848) knots 0 0 0 0 1 1 1 1
  spline S57 degree 3 poles (304.277, -10.6848) (304.4358, -11.1346) (304.7003, -11.2934) (305.5999, -11.2934) knots -1 -1 -1 -1 0 0 0 0
  spline S58 degree 3 poles (-31.4982, 6.5132) (-31.2855, 6.5132) (-31.0197, 5.931) (-31.0197, 5.6137) knots 0 0 0 0 1 1 1 1
  spline S59 degree 3 poles (-31.0197, 5.6137) (-31.0197, 5.931) (-31.2855, 6.5132) (-31.4982, 6.5132) knots -1 -1 -1 -1 0 0 0 0
  spline S60 degree 3 poles (215.3532, -11.214) (212.628, -11.214) (209.8764, -11.2405) (207.9184, -11.2934) knots 0 0 0 0 1 1 1 1
  spline S61 degree 3 poles (207.9184, -11.2934) (209.8764, -11.2405) (212.628, -11.214) (215.3532, -11.214) knots -1 -1 -1 -1 0 0 0 0
  spline S62 degree 3 poles (210.1145, -5.4725) (210.2468, -3.303) (210.2468, -1.1334) (210.1145, 1.0362) knots 0 0 0 0 1 1 1 1
  spline S63 degree 3 poles (210.1145, 1.0362) (210.2468, -1.1334) (210.2468, -3.303) (210.1145, -5.4725) knots -1 -1 -1 -1 0 0 0 0
  spline S64 degree 3 poles (99.7859, 6.5131) (100.6855, 6.4602) (101.3469, 6.4337) (102.0084, 6.4337) knots 0 0 0 0 1 1 1 1
  spline S65 degree 3 poles (102.0084, 6.4337) (101.3469, 6.4337) (100.6855, 6.4602) (99.7859, 6.5131) knots -1 -1 -1 -1 0 0 0 0
  spline S66 degree 3 poles (5.5155, -11.2142) (3.6357, -11.2142) (3.2124, -11.2935) (0.4331, -11.2935) knots 0 0 0 0 1 1 1 1
  spline S67 degree 3 poles (0.4331, -11.2935) (3.2124, -11.2935) (3.6357, -11.2142) (5.5155, -11.2142) knots -1 -1 -1 -1 0 0 0 0
  spline S68 degree 3 poles (222.4441, -10.3938) (222.4441, -10.7113) (222.1795, -11.2934) (221.9414, -11.2934) knots 0 0 0 0 1 1 1 1
  spline S69 degree 3 poles (221.9414, -11.2934) (222.1795, -11.2934) (222.4441, -10.7113) (222.4441, -10.3938) knots -1 -1 -1 -1 0 0 0 0
  spline S70 degree 3 poles (89.7317, -11.2934) (89.52, -11.3225) (89.2555, -10.7378) (89.2555, -10.4203) knots 0 0 0 0 1 1 1 1
  spline S71 degree 3 poles (89.2555, -10.4203) (89.2555, -10.7378) (89.52, -11.3225) (89.7317, -11.2934) knots -1 -1 -1 -1 0 0 0 0
  spline S72 degree 3 poles (160.2934, -11.2934) (160.0818, -11.3225) (159.7907, -10.7378) (159.7907, -10.4203) knots 0 0 0 0 1 1 1 1
  spline S73 degree 3 poles (159.7907, -10.4203) (159.7907, -10.7378) (160.0818, -11.3225) (160.2934, -11.2934) knots -1 -1 -1 -1 0 0 0 0
  spline S74 degree 3 poles (210.1145, 1.0362) (210.1145, 1.2479) (210.6966, 1.5389) (211.0141, 1.5389) knots 0 0 0 0 1 1 1 1
  spline S75 degree 3 poles (211.0141, 1.5389) (210.6966, 1.5389) (210.1145, 1.2479) (210.1145, 1.0362) knots -1 -1 -1 -1 0 0 0 0
  line L14 (99.7859, 6.5131) -> (95.7113, -4.7053)
  line L15 (95.7113, -4.7053) -> (99.7859, 6.5131)
  spline S76 degree 3 poles (89.2555, -10.4203) (89.2555, -9.9969) (90.9223, -10.0234) (90.8165, -8.9121) knots 0 0 0 0 1 1 1 1
  spline S77 degree 3 poles (90.8165, -8.9121) (90.9223, -10.0234) (89.2555, -9.9969) (89.2555, -10.4203) knots -1 -1 -1 -1 0 0 0 0
  spline S78 degree 3 poles (221.0153, -8.9386) (221.0153, -10.0763) (222.4441, -9.9969) (222.4441, -10.3938) knots 0 0 0 0 1 1 1 1
  spline S79 degree 3 poles (222.4441, -10.3938) (222.4441, -9.9969) (221.0153, -10.0763) (221.0153, -8.9386) knots -1 -1 -1 -1 0 0 0 0
  spline S80 degree 3 poles (-9.5918, 6.5131) (-6.3923, 6.328) (-4.9108, 6.4867) (-4.0362, 6.4867) knots 0 0 0 0 1 1 1 1
  spline S81 degree 3 poles (-4.0362, 6.4867) (-4.9108, 6.4867) (-6.3923, 6.328) (-9.5918, 6.5131) knots -1 -1 -1 -1 0 0 0 0
  spline S82 degree 3 poles (-23.0859, -11.2934) (-23.4287, -11.2934) (-23.6177, -10.976) (-23.7491, -10.4733) knots 0 0 0 0 1 1 1 1
  spline S83 degree 3 poles (-23.7491, -10.4733) (-23.6177, -10.976) (-23.4287, -11.2934) (-23.0859, -11.2934) knots -1 -1 -1 -1 0 0 0 0
  line L16 (309.9129, -9.6794) -> (314.8347, 4.1318)
  line L17 (314.8347, 4.1318) -> (309.9129, -9.6794)
  spline S84 degree 3 poles (-24.9921, 1.3536) (-24.9921, 4.8197) (-22.2658, 6.7775) (-17.4217, 6.7775) knots 0 0 0 0 1 1 1 1
  spline S85 degree 3 poles (-17.4217, 6.7775) (-22.2658, 6.7775) (-24.9921, 4.8197) (-24.9921, 1.3536) knots -1 -1 -1 -1 0 0 0 0
  spline S86 degree 3 poles (310.8919, -10.4203) (310.8919, -10.7378) (310.6011, -11.3225) (310.3894, -11.2934) knots 0 0 0 0 1 1 1 1
  spline S87 degree 3 poles (310.3894, -11.2934) (310.6011, -11.3225) (310.8919, -10.7378) (310.8919, -10.4203) knots -1 -1 -1 -1 0 0 0 0
  ellipse E0 centre (-60.2658, -11.5026) end of major axis (-63.0589, -11.5087) minor radius 0.2884 (-58.3, -11.2935) -> (-60.2059, -11.2142) ccw
  ellipse E1 centre (-60.2658, -11.5026) end of major axis (-63.0589, -11.5087) minor radius 0.2884 (-58.3, -11.2935) -> (-60.2059, -11.2142) ccw
  spline S88 degree 3 poles (-23.7491, -10.4733) (-23.8804, -10.0763) (-24.4347, -6.7163) (-24.4347, -6.5045) knots 0 0 0 0 1 1 1 1
  spline S89 degree 3 poles (-24.4347, -6.5045) (-24.4347, -6.7163) (-23.8804, -10.0763) (-23.7491, -10.4733) knots -1 -1 -1 -1 0 0 0 0
  line L18 (305.6267, 1.5654) -> (304.7004, 4.1318)
  line L19 (304.7004, 4.1318) -> (305.6267, 1.5654)
  spline S90 degree 3 poles (-15.6244, -7.8539) (-15.6244, -4.5467) (-24.9921, -5.1022) (-24.9921, 1.3536) knots 0 0 0 0 1 1 1 1
  spline S91 degree 3 poles (-24.9921, 1.3536) (-24.9921, -5.1022) (-15.6244, -4.5467) (-15.6244, -7.8539) knots -1 -1 -1 -1 0 0 0 0
  spline S92 degree 3 poles (-53.9628, 6.7775) (-49.3578, 6.7775) (-46.7651, 4.158) (-46.7651, -0.6308) knots 0.000005 0.000005 0.000005 0.000005 1 1 1 1
  spline S93 degree 3 poles (-46.7651, -0.6308) (-46.7651, 4.158) (-49.3578, 6.7775) (-53.9628, 6.7775) knots -1 -1 -1 -1 -0.000005 -0.000005 -0.000005 -0.000005
  spline S94 degree 3 poles (-24.4347, -6.5045) (-24.4347, -6.2927) (-23.8804, -5.7372) (-23.5601, -5.7372) knots 0 0 0 0 1 1 1 1
  spline S95 degree 3 poles (-23.5601, -5.7372) (-23.8804, -5.7372) (-24.4347, -6.2927) (-24.4347, -6.5045) knots -1 -1 -1 -1 0 0 0 0
  spline S96 degree 3 poles (-17.8446, -9.6531) (-16.5759, -9.6531) (-15.6244, -8.8858) (-15.6244, -7.8539) knots 0 0 0 0 1 1 1 1
  spline S97 degree 3 poles (-15.6244, -7.8539) (-15.6244, -8.8858) (-16.5759, -9.6531) (-17.8446, -9.6531) knots -1 -1 -1 -1 0 0 0 0
  ellipse E2 centre (-60.1459, -11.5026) end of major axis (-62.939, -11.4965) minor radius 0.2884 (-60.2059, -11.2142) -> (-62.1118, -11.2935) ccw
  ellipse E3 centre (-60.1459, -11.5026) end of major axis (-62.939, -11.4965) minor radius 0.2884 (-60.2059, -11.2142) -> (-62.1118, -11.2935) ccw
  line L20 (215.6707, 4.1583) -> (215.6707, -1.2921)
  line L21 (215.6707, -1.2921) -> (215.6707, 4.1583)
  spline S98 degree 3 poles (-8.5087, -5.8961) (-8.5087, -3.5677) (-6.8685, -1.9008) (-4.0362, -1.0807) knots 0 0 0 0 1 1 1 1
  spline S99 degree 3 poles (-4.0362, -1.0807) (-6.8685, -1.9008) (-8.5087, -3.5677) (-8.5087, -5.8961) knots -1 -1 -1 -1 0 0 0 0
  spline S100 degree 3 poles (19.7498, -9.7058) (17.3937, -9.7058) (16.2828, -7.3512) (16.2828, -2.3771) knots -1 -1 -1 -1 0 0 0 0
  spline S101 degree 3 poles (19.7498, -9.7058) (17.3937, -9.7058) (16.2828, -7.3512) (16.2828, -2.3771) knots -1 -1 -1 -1 0 0 0 0
  spline S102 degree 3 poles (92.1394, 6.4337) (93.7005, 6.4337) (95.288, 6.4602) (95.6848, 6.5131) knots 0 0 0 0 1 1 1 1
  spline S103 degree 3 poles (95.6848, 6.5131) (95.288, 6.4602) (93.7005, 6.4337) (92.1394, 6.4337) knots -1 -1 -1 -1 0 0 0 0
  line L22 (95.7113, -4.7053) -> (94.7323, 4.1583)
  line L23 (94.7323, 4.1583) -> (95.7113, -4.7053)
  spline S104 degree 3 poles (211.0141, 1.5389) (211.8078, 1.5389) (211.6491, -1.1863) (213.8186, -1.2392) knots 0 0 0 0 1 1 1 1
  spline S105 degree 3 poles (213.8186, -1.2392) (211.6491, -1.1863) (211.8078, 1.5389) (211.0141, 1.5389) knots -1 -1 -1 -1 0 0 0 0
  spline S106 degree 3 poles (15.2526, 12.1222) (19.1944, 12.0165) (22.2105, 7.307) (24.1426, 7.307) knots 0 0 0 0 1 1 1 1
  spline S107 degree 3 poles (24.1426, 7.307) (22.2105, 7.307) (19.1944, 12.0165) (15.2526, 12.1222) knots -1 -1 -1 -1 0 0 0 0
  line L24 (89.3877, 4.1583) -> (90.8165, -8.9121)
  line L25 (90.8165, -8.9121) -> (89.3877, 4.1583)
  spline S108 degree 3 poles (0.4331, -11.2935) (-5.0695, -11.2935) (-8.5087, -9.2826) (-8.5087, -5.8961) knots 0 0 0 0 1 1 1 1
  spline S109 degree 3 poles (-8.5087, -5.8961) (-8.5087, -9.2826) (-5.0695, -11.2935) (0.4331, -11.2935) knots -1 -1 -1 -1 0 0 0 0
  spline S110 degree 3 poles (96.1875, 5.6135) (96.1875, 5.2166) (94.6265, 5.296) (94.7323, 4.1583) knots 0 0 0 0 1 1 1 1
  spline S111 degree 3 poles (94.7323, 4.1583) (94.6265, 5.296) (96.1875, 5.2166) (96.1875, 5.6135) knots -1 -1 -1 -1 0 0 0 0
  line L26 (221.0153, -8.9386) -> (221.0153, 4.1583)
  line L27 (221.0153, 4.1583) -> (221.0153, -8.9386)
  spline S112 degree 3 poles (89.3877, 4.1583) (89.2819, 5.296) (88.0913, 5.2166) (88.0913, 5.6135) knots 0 0 0 0 1 1 1 1
  spline S113 degree 3 poles (88.0913, 5.6135) (88.0913, 5.2166) (89.2819, 5.296) (89.3877, 4.1583) knots -1 -1 -1 -1 0 0 0 0
  line L28 (215.6707, -1.2921) -> (213.8186, -1.2392)
  line L29 (213.8186, -1.2392) -> (215.6707, -1.2921)
  ellipse E4 centre (19.5885, -1.7408) end of major axis (19.5885, -11.5568) minor radius 8.5372 (19.5885, -11.5568) -> (26.2098, 4.4555) ccw
  ellipse E5 centre (19.5885, -1.7408) end of major axis (19.5885, -11.5568) minor radius 8.5372 (19.5885, -11.5568) -> (26.2098, 4.4555) ccw
  spline S114 degree 3 poles (-10.096, 5.6134) (-10.096, 5.9308) (-9.8034, 6.5131) (-9.5918, 6.5131) knots 0 0 0 0 1 1 1 1
  spline S115 degree 3 poles (-9.5918, 6.5131) (-9.8034, 6.5131) (-10.096, 5.9308) (-10.096, 5.6134) knots -1 -1 -1 -1 0 0 0 0
  spline S116 degree 3 poles (95.6848, 6.5131) (95.8965, 6.5395) (96.1875, 5.931) (96.1875, 5.6135) knots 0 0 0 0 1 1 1 1
  spline S117 degree 3 poles (96.1875, 5.6135) (96.1875, 5.931) (95.8965, 6.5395) (95.6848, 6.5131) knots -1 -1 -1 -1 0 0 0 0
  spline S118 degree 3 poles (222.4441, 5.64) (222.4441, 5.2166) (221.0153, 5.296) (221.0153, 4.1583) knots 0 0 0 0 1 1 1 1
  spline S119 degree 3 poles (221.0153, 4.1583) (221.0153, 5.296) (222.4441, 5.2166) (222.4441, 5.64) knots -1 -1 -1 -1 0 0 0 0
  spline S120 degree 3 poles (-71.625, -11.231) (-71.7664, -11.1349) (-71.9088, -10.861) (-71.9703, -10.6166) knots 0.15171 0.15171 0.15171 0.15171 0.790921 0.790921 0.790921 0.790921
  spline S121 degree 3 poles (-71.9703, -10.6166) (-71.9088, -10.861) (-71.7664, -11.1349) (-71.625, -11.231) knots -0.790921 -0.790921 -0.790921 -0.790921 -0.15171 -0.15171 -0.15171 -0.15171
  line L30 (-74.6506, 2.4388) -> (-70.6626, -9.3268)
  line L31 (-70.6626, -9.3268) -> (-74.6506, 2.4388)
  line L32 (2.7113, -9.4149) -> (1.3605, -9.4149)
  spline S122 degree 3 poles (1.3605, -9.4149) (-1.285, -9.4149) (-2.6606, -8.0125) (-2.6606, -5.949) knots -1 -1 -1 -1 0 0 0 0
  spline S123 degree 3 poles (-2.6606, -5.949) (-2.6606, -3.8323) (-1.2321, -2.4299) (1.4134, -2.4299) knots -1 -1 -1 -1 0 0 0 0
  spline S124 degree 3 poles (1.4134, -2.4299) (1.8367, -2.4299) (2.7113, -2.377) (2.7113, -3.0383) knots -1 -1 -1 -1 0 0 0 0
  line L33 (2.7113, -3.0383) -> (2.7113, -9.4149)
  spline S125 degree 3 poles (8.0583, 4.1848) (8.0583, 5.2959) (9.5118, 5.2165) (9.5118, 5.6398) knots -1 -1 -1 -1 0 0 0 0
  spline S126 degree 3 poles (9.5118, 5.6398) (9.5118, 5.9573) (9.2223, 6.5131) (9.0107, 6.5131) knots -1 -1 -1 -1 0 0 0 0
  spline S127 degree 3 poles (9.0107, 6.5131) (7.9525, 6.4602) (6.6827, 6.4338) (5.3848, 6.4338) knots -1 -1 -1 -1 0 0 0 0
  spline S128 degree 3 poles (5.3848, 6.4338) (4.087, 6.4338) (2.7891, 6.4602) (1.7558, 6.5131) knots -1 -1 -1 -1 0 0 0 0
  spline S129 degree 3 poles (1.7558, 6.5131) (1.5442, 6.5131) (1.2548, 5.9573) (1.2548, 5.6398) knots -1 -1 -1 -1 0 0 0 0
  spline S130 degree 3 poles (1.2548, 5.6398) (1.2548, 5.2165) (2.7113, 5.2959) (2.7113, 4.1848) knots -1 -1 -1 -1 0 0 0 0
  line L34 (2.7113, 4.1848) -> (2.7113, -0.5248)
  line L35 (2.7113, -0.5248) -> (0.9622, -0.5248)
  line L36 (0.9622, -0.5248) -> (-2.1844, 4.1319)
  spline S131 degree 3 poles (-2.1844, 4.1319) (-3.3764, 5.8779) (-2.3431, 6.4867) (-4.0362, 6.4867) knots -1 -1 -1 -1 0 0 0 0
  spline S132 degree 3 poles (-4.0362, 6.4867) (-4.9108, 6.4867) (-6.3923, 6.328) (-9.5918, 6.5131) knots -1 -1 -1 -1 0 0 0 0
  spline S133 degree 3 poles (-9.5918, 6.5131) (-9.8034, 6.5131) (-10.096, 5.9308) (-10.096, 5.6134) knots -1 -1 -1 -1 0 0 0 0
  spline S134 degree 3 poles (-10.096, 5.6134) (-10.096, 5.2165) (-8.851, 5.1107) (-8.269, 4.1319) knots -1 -1 -1 -1 0 0 0 0
  spline S135 degree 3 poles (-8.269, 4.1319) (-6.9463, 1.9358) (-6.0748, -0.3396) (-4.0362, -1.0807) knots -1 -1 -1 -1 0 0 0 0
  spline S136 degree 3 poles (-4.0362, -1.0807) (-6.8685, -1.9008) (-8.5087, -3.5677) (-8.5087, -5.8961) knots -1 -1 -1 -1 0 0 0 0
  spline S137 degree 3 poles (-8.5087, -5.8961) (-8.5087, -9.2826) (-5.0695, -11.2935) (0.4331, -11.2935) knots -1 -1 -1 -1 0 0 0 0
  spline S138 degree 3 poles (0.4331, -11.2935) (3.2124, -11.2935) (3.6357, -11.2142) (5.5155, -11.2142) knots -1 -1 -1 -1 0 0 0 0
  spline S139 degree 3 poles (5.5155, -11.2142) (6.6827, -11.2142) (7.9525, -11.2406) (9.0107, -11.2935) knots -1 -1 -1 -1 0 0 0 0
  spline S140 degree 3 poles (9.0107, -11.2935) (9.2223, -11.3225) (9.5118, -10.738) (9.5118, -10.4202) knots -1 -1 -1 -1 0 0 0 0
  spline S141 degree 3 poles (9.5118, -10.4202) (9.5118, -9.9969) (8.0583, -10.0763) (8.0583, -8.9652) knots -1 -1 -1 -1 0 0 0 0
  line L37 (8.0583, -8.9652) -> (8.0583, 4.1848)
  spline S142 degree 5 poles (-71.9703, -10.6166) (-71.967, -10.6087) (-71.9463, -10.562) (-71.8986, -10.4733) (-71.821, -10.3613) (-71.7201, -10.2417) (-71.6088, -10.1255) (-71.5378, -10.0556) (-71.5166, -10.0352) knots 0.479543 0.479543 0.479543 0.479543 0.479543 0.479543 0.5 0.6 0.7 0.740882 0.740882 0.740882 0.740882 0.740882 0.740882
  spline S143 degree 5 poles (-71.5166, -10.0352) (-71.5378, -10.0556) (-71.6088, -10.1255) (-71.7201, -10.2417) (-71.821, -10.3613) (-71.8986, -10.4733) (-71.9463, -10.562) (-71.967, -10.6087) (-71.9703, -10.6166) knots -0.740882 -0.740882 -0.740882 -0.740882 -0.740882 -0.740882 -0.7 -0.6 -0.5 -0.479543 -0.479543 -0.479543 -0.479543 -0.479543 -0.479543
  spline S144 degree 3 poles (159.7907, -10.4203) (159.7907, -10.0234) (161.2459, -10.0763) (161.2459, -8.965) knots 0 0 0 0 1 1 1 1